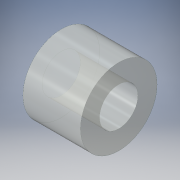
# Autodesk Inventor part: bearing tube_xw
Saved by Autodesk Inventor 2016 (Build 200138000, 138)
## iProperties
Created: 2015-06-09
Part Number: bearing tube_xw
Material: Generic
Document SubType Name: Modeling
Designer: 121767
Density: 1 g/cm^3
Appearance: Clear
Author: 121767
Autodesk Inventor part; units mm, degrees
ref_plane "YZ Plane" through (0, 0, 0) normal (1, 0, 0) x (0, 1, 0)
ref_plane "XZ Plane" through (0, 0, 0) normal (0, 1, 0) x (-1, 0, 0)
ref_plane "XY Plane" through (0, 0, 0) normal (0, 0, 1) x (1, 0, 0)
sketch "Sketch1" plane through (0, 0, 0) normal (1, 0, 0) x (0, 1, 0)
  circle A0 centre (0, 0) radius 0.5
  circle A1 centre (0, 0) radius 0.25
  dimension "d13" = 0.5
  dimension "d14" = 1
  constraints: 2 centre point, 2 coincident
  measures "d13" diameter of A1
  measures "d14" diameter of A0
extrude "Extrusion2" add sketch "Sketch1" along normal blind 0.75
body "Solid2"
